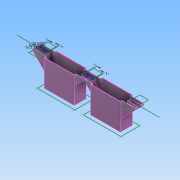
# Autodesk Inventor part: ViaductPillarsUnit_S
Saved by Autodesk Inventor 2021 (Build 250183000, 183)
## iProperties
Created: 2021-03-15
Part Number: ViaductPillarsUnit_S
Material: 一般
Document SubType Name: Modeling
Designer: kumagai
Density: 1 g/cm^3
Appearance: 滑らか - 紫
Author: kumagai
Autodesk Inventor part; units mm, degrees
derived "ViaductPillarsUnitIC.ipt"
feature "ソリッド1::ViaductPillarsUnitIC.ipt" [suppressed]
sketch "SupportBase" plane through (0, 0, 0) normal (0, -1, 0) x (1, 0, 0)
  line L0 (-48.75, 11) -> (-48.75, -11)
  line L1 (-48.75, -11) -> (-5, -11)
  line L2 (-48.75, 11) -> (-5, 11)
  line L3 (-5, 11) -> (-5, -11)
  line L4 (5, 11) -> (5, -11)
  line L5 (5, -11) -> (48.75, -11)
  line L6 (48.75, -11) -> (48.75, 11)
  line L7 (5, 11) -> (48.75, 11)
sketch "SupportTarget" plane through (0, 31, 0) normal (0, -1, 0) x (1, 0, 0)
  line L0 (48.75, 11) -> (58.75, 11)
  line L1 (48.75, 11) -> (48.75, -11)
  line L2 (58.75, -11) -> (48.75, -11)
  line L3 (58.75, -11) -> (58.75, 11)
  line L4 (-5, 11) -> (5, 11)
  line L5 (-5, 11) -> (-5, -11)
  line L6 (5, -11) -> (-5, -11)
  line L7 (5, -11) -> (5, 11)
  line L8 (-58.75, 11) -> (-58.75, -11)
  line L9 (-48.75, -11) -> (-58.75, -11)
  line L10 (-48.75, -11) -> (-48.75, 11)
  line L11 (-58.75, 11) -> (-48.75, 11)
ref_plane "作業平面1" through (-48.75, 0, 11) normal (0, 1, 0) x (1, 0, 0)
ref_plane "作業平面2" through (-48.75, 31, -11) normal (0, 1, 0) x (0, 0, 1)
sketch "スケッチ4" plane through (-48.75, 0, 11) normal (0, 1, 0) x (1, 0, 0)
  line L0 (4.375, 4) -> (39.375, 4)
  line L1 (39.375, 4) -> (39.375, 18)
  line L2 (39.375, 18) -> (4.375, 18)
  line L3 (4.375, 18) -> (4.375, 4)
  line L4 (48.75, 26.4) -> (48.75, -4.4) projected
  line L5 (131, 11) -> (-33.5, 11) projected
  line L6 (93.125, 4) -> (58.125, 4)
  line L7 (58.125, 4) -> (58.125, 18)
  line L8 (58.125, 18) -> (93.125, 18)
  line L9 (93.125, 18) -> (93.125, 4)
  line L10 (0, 0) -> (0, 22) projected
  line L11 (43.75, 0) -> (43.75, 22) projected
  line L12 (0, 22) -> (43.75, 22) projected
  line L13 (0, 0) -> (43.75, 0) projected
  point P0 (48.75, 11)
  dimension "d13" = 35
  dimension "d16" = 14
  dimension "d87" = 4.375
  dimension "d88" = 4.375
  dimension "d89" = 4
  dimension "d91" = 4
  constraints: 16 end point, 4 symmetric about line
  measures "d13" distance between parallel lines of L1 L3
  measures "d16" distance between parallel lines of L2 L0
  measures "d87" distance between parallel lines of L10 L3
  measures "d88" distance between parallel lines of L11 L1
  measures "d89" distance between parallel lines of L12 L2
  measures "d91" distance between parallel lines of L13 L0
ref_plane "作業平面3" through (-48.75, 30.8, -11) normal (0, 1, 0) x (0, 0, 1)
extrude "押し出し1" add sketch "スケッチ4" along normal up to surface (30.8 mm away) contours L3 L5 L1 L0 | L3 L2 L1 L5 | L9 L6 L7 L5 | L5 L7 L8 L9
sketch "スケッチ5" plane through (-48.75, 30.8, -11) normal (0, 1, 0) x (0, 0, 1)
  line L0 (-4.4, 48.75) -> (26.4, 48.75) projected
  line L1 (11, 132.4) -> (11, -34.9) projected
  line L2 (0, 0) -> (22, 0) projected
  line L3 (22, 43.75) -> (0, 43.75) projected
  line L4 (0, 53.75) -> (22, 53.75) projected
  line L5 (22, 97.5) -> (0, 97.5) projected
  line L6 (22, -10) -> (0, -10) projected
  line L7 (0, 107.5) -> (22, 107.5) projected
  line L8 (6, -11) -> (16, -11)
  line L9 (16, -11) -> (16, 108.5)
  line L10 (16, 108.5) -> (6, 108.5)
  line L11 (6, 108.5) -> (6, -11)
  dimension "d93" = 6
  dimension "d95" = 1
  dimension "d96" = 1
  constraints: 8 end point, 1 vertical, 1 other
  measures "d93" distance from line of L11 L6.end
  measures "d95" distance between parallel lines of L6 L8
  measures "d96" distance between parallel lines of L7 L10
extrude "押し出し2" add sketch "スケッチ5" against normal blind 2
draft "面の勾配3" angle 45 pull direction (-1, 0, 0) faces at (-49.5, 28.8, -1.6667) fixed edges at (-59.75, 28.8, 0)
draft "面の勾配4" angle 45 pull direction (1, 0, 0) faces at (54.625, 28.8, 1.6667) fixed edges at (59.75, 28.8, 0)
sketch "スケッチ7" plane through (4.375, 30.8, 5) normal (0, 0, -1) x (-1, 0, 0)
  line L0 (13.75, -30.8) -> (13.75, 0) projected
  line L1 (-5, -30.8) -> (-5, 0) projected
  line L2 (13.75, -2) -> (-5, -2) projected
  line L3 (4.375, -2) -> (13.75, -11.375)
  line L4 (13.75, -2) -> (13.75, -10.0248)
  line L5 (13.75, -2) -> (4.375, -2)
  line L6 (4.375, -2) -> (-5, -2)
  line L7 (-5, -2) -> (-5, -11.375)
  line L8 (-5, -11.375) -> (4.375, -2)
  dimension "d102" = 45
  dimension "d103" = 45
  constraints: 12 end point, 5 point on line, 2 midpoint
  measures "d102" angle of L2 L3
  measures "d103" angle of L2 L8
extrude "押し出し3" add sketch "スケッチ7" along normal up to surface (10 mm away)
sketch "スケッチ8" plane through (-48.75, 30.8, -11) normal (0, 1, 0) x (0, 0, 1)
  line L0 (11, 131.2) -> (11, -34.7) projected
  line L1 (12.6667, -11) -> (9.3333, -11)
  line L2 (9.3333, -11) -> (9.3333, 1)
  line L3 (9.3333, 1) -> (12.6667, 1)
  line L4 (12.6667, 1) -> (12.6667, -11)
  line L5 (12.6667, 42.75) -> (9.3333, 42.75)
  line L6 (9.3333, 42.75) -> (9.3333, 54.75)
  line L7 (9.3333, 54.75) -> (12.6667, 54.75)
  line L8 (12.6667, 54.75) -> (12.6667, 42.75)
  line L9 (16, -11) -> (16, 4.375) projected
  line L10 (6, 4.375) -> (6, -11) projected
  line L11 (22, -10) -> (0, -10) projected
  line L12 (0, 0) -> (22, 0) projected
  line L13 (22, 43.75) -> (0, 43.75) projected
  line L14 (0, 53.75) -> (22, 53.75) projected
  dimension "d107" = 3.3333
  dimension "d108" = 3.3333
  dimension "d109" = 3.3333
  dimension "d113" = 1
  dimension "d114" = 1
  dimension "d115" = 1
  dimension "d116" = 1
  constraints: 16 end point, 2 collinear, 2 point on line
  measures "d107" distance between parallel lines of L4 L9
  measures "d108" distance between parallel lines of L2 L4
  measures "d109" distance between parallel lines of L10 L2
  measures "d113" distance between parallel lines of L1 L11
  measures "d114" distance between parallel lines of L3 L12
  measures "d115" distance between parallel lines of L5 L13
  measures "d116" distance between parallel lines of L7 L14
extrude "押し出し4" cut sketch "スケッチ8" along normal through all both and the other way through all contours L3 L4 L12 L0 | L0 L12 L2 L3 | L12 L4 L11 L0 | L0 L11 L2 L12 | L11 L4 L1 L0 | L0 L1 L2 L11
mirror "ミラー1" about plane through (0, 0, 0) normal (1, 0, 0) of "押し出し4"
extrude "押し出し6" cut sketch "スケッチ8" against normal through all contours L7 L8 L14 L0 | L0 L14 L6 L7 | L14 L8 L13 L0 | L0 L13 L6 L14 | L13 L8 L5 L0 | L0 L5 L6 L13
shell "シェル2" thickness 0.5 removed faces 1 at (32.7083, 30.8, -1.6667)
equation "\"d87\" = d88"
equation "\"d89\" = d91"
equation "\"d31\" = SupAngle"
equation "\"d32\" = SupAngle"
equation "\"d102\" = SupAngle"
equation "\"d103\" = SupAngle"
equation "\"d107\" = d109"
equation "\"d108\" = d109"
equation "\"d64\" = SupportRib"
equation "\"d19\" = -SupportGap"
equation "\"VBW\" = 8"
equation "\"SupAngle\" = 45deg"
equation "\"SupportRib\" = 0.5"
equation "\"SupportGap\" = 0.2"
